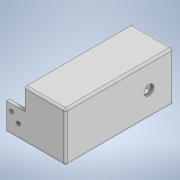
# Autodesk Inventor part: PSUCover
Saved by Autodesk Inventor 2020 (Build 240168000, 168)
## iProperties
Created: 2020-01-14
Part Number: PSUCover
Material: Generic
Document SubType Name: Modeling
Designer: PAB
Density: 1 g/cm^3
Appearance: Default
Author: PAB
Autodesk Inventor part; units mm, degrees
ref_plane "YZ Plane" through (0, 0, 0) normal (1, 0, 0) x (0, 1, 0)
ref_plane "XZ Plane" through (0, 0, 0) normal (0, 1, 0) x (-1, 0, 0)
ref_plane "XY Plane" through (0, 0, 0) normal (0, 0, 1) x (1, 0, 0)
sketch "Sketch1" plane through (0, 0, 0) normal (0, 1, 0) x (-1, 0, 0)
  line L0 (30, 55) -> (-30, 55)
  line L1 (-30, 55) -> (-30, -55)
  line L2 (-30, -55) -> (30, -55)
  line L3 (30, -55) -> (30, 55)
  point P0 (0, 0)
  dimension "d0" = 60
  dimension "d1" = 110
  constraints: 8 end point, 2 parallel, 1 horizontal, 1 perpendicular
  measures "d0" distance of L2.end L1.end
  measures "d1" distance of L1.end L0.end
extrude "Extrusion1" add sketch "Sketch1" along normal blind 3
sketch "Sketch2" plane through (0, 3, 0) normal (0, 1, 0) x (1, 0, 0)
  line L0 (30, 55) -> (-30, 55) projected
  line L1 (30, 55) -> (-11, 55)
  line L2 (-11, 55) -> (-11, 52)
  line L3 (-11, 52) -> (30, 52)
  line L4 (30, 52) -> (30, 55)
  line L5 (-30, -55) -> (30, -55) projected
  line L6 (30, -55) -> (-11, -55)
  line L7 (-11, -55) -> (-11, -52)
  line L8 (-11, -52) -> (30, -52)
  line L9 (30, -52) -> (30, -55)
  line L10 (30, 52) -> (27, 52)
  line L11 (27, 52) -> (27, -52)
  line L12 (27, -52) -> (30, -52)
  line L13 (30, -52) -> (30, 52)
  point P0 (0, 0)
  dimension "d4" = 41
  dimension "d5" = 3
  dimension "d6" = 41
  dimension "d7" = 3
  dimension "d8" = 3
  constraints: 24 end point, 6 parallel, 3 horizontal, 3 perpendicular, 1 point on line
  measures "d4" distance of L3.end L2.end
  measures "d5" distance of L2.end L1.end
  measures "d6" distance of L7.end L8.end
  measures "d7" distance of L6.end L7.end
  measures "d8" distance of L12.end L11.end
extrude "Extrusion2" add sketch "Sketch2" along normal blind 47
sketch "Sketch3" plane through (0, 3, 0) normal (0, 1, 0) x (1, 0, 0)
  line L0 (27, -52) -> (-11, -52) projected
  line L1 (-30, -55) -> (30, -55) projected
  line L2 (-11, -52) -> (-30, -52)
  line L3 (-30, -52) -> (-30, -55)
  line L4 (-30, -55) -> (-11, -55)
  line L5 (-11, -55) -> (-11, -52)
  line L6 (30, 55) -> (-30, 55) projected
  line L7 (-30, 55) -> (-30, -55) projected
  line L8 (-11, 55) -> (-30, 55)
  line L9 (-30, 55) -> (-30, 52)
  line L10 (-30, 52) -> (-11, 52)
  line L11 (-11, 52) -> (-11, 55)
  line L12 (-30, 52) -> (-27, 52)
  line L13 (-27, 52) -> (-27, -52)
  line L14 (-27, -52) -> (-30, -52)
  line L15 (-30, -52) -> (-30, 52)
  point P0 (0, 0)
  dimension "d11" = 3
  dimension "d12" = 3
  constraints: 24 end point, 6 parallel, 4 point on line, 3 horizontal, 3 perpendicular
  measures "d11" distance of L9.end L8.end
  measures "d12" distance of L13.end L14.end
extrude "Extrusion3" add sketch "Sketch3" along normal blind 25
sketch "Sketch4" plane through (0, 0, 0) normal (0, -1, 0) x (1, 0, 0)
  line L0 (14, 24) -> (-14, 24)
  line L1 (-14, 24) -> (-14, -24)
  line L2 (-14, -24) -> (14, -24)
  line L3 (14, -24) -> (14, 24)
  circle A0 centre (20, 0) radius 2
  circle A1 centre (-20, 0) radius 2
  point P0 (0, 0)
  dimension "d15" = 28
  dimension "d16" = 48
  dimension "d17" = 4
  dimension "d18" = 4
  constraints: 8 end point, 2 centre point, 2 parallel, 1 horizontal, 1 perpendicular
  measures "d15" distance of L2.end L1.end
  measures "d16" distance of L1.end L0.end
  measures "d17" diameter of A0
  measures "d18" diameter of A1
extrude "Extrusion4" cut sketch "Sketch4" against normal blind 3
sketch "Sketch5" plane through (-30, 0, 55) normal (0, 0, 1) x (1, 0, 0)
  circle A0 centre (12, 14) radius 2
  circle A1 centre (5, 21) radius 2
  point P0 (30, 0)
  dimension "d21" = 4
  dimension "d22" = 4
  constraints: 2 centre point
  measures "d21" diameter of A0
  measures "d22" diameter of A1
extrude "Extrusion5" cut sketch "Sketch5" against normal blind 110
sketch "Sketch6" plane through (30, 0, 55) normal (1, 0, 0) x (0, 0, -1)
  circle A0 centre (85, 25) radius 5
  point P0 (55, 0)
  dimension "d25" = 10
  constraints: 1 centre point
  measures "d25" diameter of A0
extrude "Extrusion6" cut sketch "Sketch6" against normal blind 3
sketch "Sketch7" plane through (30, 0, 55) normal (1, 0, 0) x (0, 0, -1)
  line L0 (0, 0) -> (0, 50) projected
  line L1 (110, 28) -> (110, 50) projected
  line L2 (0, 50) -> (110, 50)
  line L3 (110, 50) -> (110, 47)
  line L4 (110, 47) -> (0, 47)
  line L5 (0, 47) -> (0, 50)
  point P0 (55, 0)
  dimension "d28" = 3
  constraints: 8 end point, 2 parallel, 1 horizontal, 1 perpendicular, 1 point on line
  measures "d28" distance of L2.end L3.end
extrude "Extrusion7" add sketch "Sketch7" against normal blind 41
sketch "Sketch8" plane through (0, 28, 0) normal (0, 1, 0) x (1, 0, 0)
  line L0 (27, 52) -> (-27, 52) projected
  line L1 (-27, 52) -> (-30, 52)
  line L2 (-30, 52) -> (-30, -52)
  line L3 (-30, -52) -> (-27, -52)
  line L4 (-27, -52) -> (-27, 52)
  point P0 (0, 0)
  dimension "d31" = 3
  dimension "d32" = 104
  constraints: 8 end point, 2 parallel, 1 horizontal, 1 perpendicular
  measures "d31" distance of L3.end L2.end
  measures "d32" distance of L2.end L1.end
extrude "Extrusion8" cut sketch "Sketch8" against normal blind 20
fillet "Fillet1" radius 2 8 edges at (9.5, 50, -55) (9.5, 50, 55) (30, 50, 0) (30, 25, -55) (0, 0, -55) (0, 0, 55) (30, 25, 55) (30, 0, 0)
sketch "Sketch9" plane through (27, 3, 52) normal (0, 0, -1) x (-1, 0, 0)
  circle A0 centre (52, 18) radius 2 projected
  circle A1 centre (52, 18) radius 4
  circle A2 centre (45, 11) radius 2 projected
  circle A3 centre (45, 11) radius 4
  point P0 (27, -3)
  dimension "d36" = 8
  dimension "d37" = 8
  constraints: 2 centre point, 2 coincident
  measures "d36" diameter of A1
  measures "d37" diameter of A3
extrude "Extrusion9" add sketch "Sketch9" along normal blind 3 contours A0 | A1 | A2 | A3
sketch "Sketch10" plane through (-25, 21, 49) normal (0, 0, -1) x (-1, 0, 0)
  circle A0 centre (0, 0) radius 2 projected
  circle A1 centre (0, 0) radius 3
  circle A2 centre (-7, -7) radius 2 projected
  circle A3 centre (-7, -7) radius 3
  point P0 (-25, -21)
  dimension "d40" = 6
  dimension "d41" = 6
  constraints: 2 centre point, 2 coincident
  measures "d40" diameter of A1
  measures "d41" diameter of A3
extrude "Extrusion10" cut sketch "Sketch10" against normal blind 3 contours A0 | A1 | A2 | A3
mirror "Mirror1" about plane through (0, 0, 0) normal (0, 0, 1) of "Extrusion10", "Extrusion9"
sketch "Sketch11" plane through (0, 3, 0) normal (0, 1, 0) x (1, 0, 0)
  circle A0 centre (20, 0) radius 2 projected
  circle A1 centre (20, 0) radius 3
  circle A2 centre (20, 0) radius 4
  circle A3 centre (-20, 0) radius 2 projected
  circle A4 centre (-20, 0) radius 3
  circle A5 centre (-20, 0) radius 4
  point P0 (0, 0)
  dimension "d44" = 6
  dimension "d45" = 8
  dimension "d46" = 6
  dimension "d47" = 8
  constraints: 4 centre point, 4 coincident
  measures "d44" diameter of A1
  measures "d45" diameter of A2
  measures "d46" diameter of A4
  measures "d47" diameter of A5
extrude "Extrusion11" add sketch "Sketch11" along normal blind 3 contours A2 | A5
sketch "Sketch12" plane through (-27, 3, -52) normal (0, 0, 1) x (1, 0, 0)
  line L0 (21, 39.5) -> (11, 39.5)
  line L1 (11, 39.5) -> (11, 36.5)
  line L2 (11, 36.5) -> (21, 36.5)
  line L3 (21, 36.5) -> (21, 39.5)
  point P0 (27, -3)
  dimension "d50" = 10
  dimension "d51" = 3
  constraints: 8 end point, 2 parallel, 1 horizontal, 1 perpendicular
  measures "d50" distance of L2.end L1.end
  measures "d51" distance of L1.end L0.end
extrude "Extrusion12" add sketch "Sketch12" along normal blind 3
sketch "Sketch13" plane through (0, 50, 0) normal (0, 1, 0) x (1, 0, 0)
  line L0 (-6, 49) -> (-16, 49) projected
  line L1 (-11, 52) -> (-11, -52) projected
  line L2 (-6, 49) -> (-11, 49)
  line L3 (-11, 49) -> (-11, 52)
  line L4 (-11, 52) -> (-6, 52)
  line L5 (-6, 52) -> (-6, 49)
  point P0 (0, 0)
  dimension "d54" = 3
  constraints: 8 end point, 2 parallel, 1 horizontal, 1 perpendicular
  measures "d54" distance of L2.end L1.start
extrude "Extrusion13" add sketch "Sketch13" against normal blind 10
body "Solid1"
